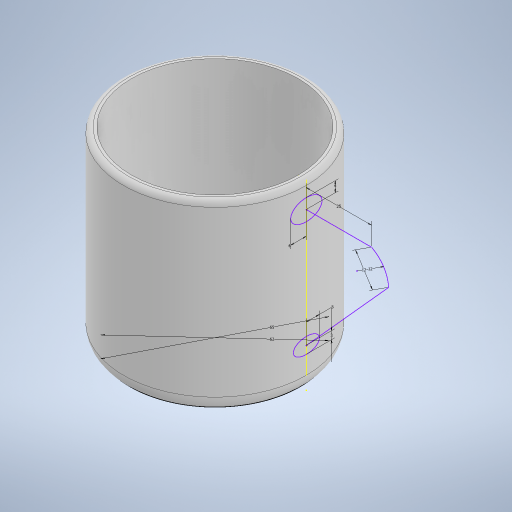
# Autodesk Inventor part: Taza Juan Molina
Saved by Autodesk Inventor 2024 (Build 280153000, 153)
## iProperties
Created: 2024-02-24
Part Number: Taza Juan Molina
Material: Genérico
Document SubType Name: Modeling
Designer: jlmol
Density: 1 g/cm^3
Appearance: Valor por defecto
Author: jlmol
Autodesk Inventor part; units mm, degrees
ref_plane "XZ Plane" through (0, 0, 0) normal (0, 1, 0) x (-1, 0, 0)
sketch "Boceto1" plane through (0, 0, 0) normal (0, 0, 1) x (1, 0, 0)
  line L0 (0, 0) -> (-32.5, 0)
  line L1 (0, 0) -> (0, 70)
  line L2 (0, 70) -> (-35, 70)
  line L3 (-35, 70) -> (-35, 5)
  arc A0 (-35, 5) -> (-32.5, 0) centre (-28.75, 5) ccw
  dimension "d0" = 32.5
  dimension "d1" = 70
  dimension "d2" = 35
  dimension "d3" = 65
  constraints: 8 end point, 2 perpendicular, 2 point on circle, 1 centre point, 1 horizontal, 1 tangent, 1 vertical
  measures "d0" distance of L0.start L0.end
  measures "d1" distance of L0.start L1.end
  measures "d2" distance of L1.end L2.end
  measures "d3" distance of L2.end L3.end
revolve "Revolución1" add sketch "Boceto1" angle 360 about axis through (0, 0, 0) along (0, 1, 0)
shell "Vaciado1" thickness 3 removed faces 1 at (-0.2748, 70, -9.3581)
sketch "Boceto2" plane through (0, 0, 0) normal (0, 0, 1) x (1, 0, 0)
  line L0 (35, 5) -> (35, 70) projected
  line L1 (32, 5) -> (32, 70) projected
  line L2 (35, 60.0697) -> (60, 60.0697)
  arc A0 (66.5079, 49.9877) -> (60, 60.0697) centre (54.5227, 49.3927) ccw
  line L3 (66.5079, 49.9877) -> (35, 15)
  point P0 (0, 0)
  dimension "d10" = 25
  dimension "d11" = 12
  dimension "d12" = 12
  constraints: 4 end point, 2 point on circle, 2 point on line, 1 centre point, 1 horizontal
  measures "d10" distance of L2.start L2.end
  measures "d11" distance of L2.end L3.start
  measures "d12" radius of A0
ref_plane "Plano de trabajo1" through (35, 60.0697, 0) normal (1, 0, 0) x (0, 1, 0)
sketch "Boceto3" plane through (35, 60.0697, 0) normal (1, 0, 0) x (0, 1, 0)
  ellipse E0 centre (0, 0) end of major axis (-4, 0) minor radius 6
  point P0 (-60.0697, 0)
  dimension "d14" = 4
  dimension "d15" = 6
  constraints: 2 other
ref_plane "Plano de trabajo10" through (35, 15, 0) normal (1, 0, 0) x (0, 1, 0)
sketch "Boceto8" plane through (35, 15, 0) normal (1, 0, 0) x (0, 1, 0)
  ellipse E0 centre (0, 0) end of major axis (-3, 0) minor radius 5
  point P0 (-15, 0)
  dimension "d23" = 5
  dimension "d24" = 3
  constraints: 2 other
fillet "Empalme1" radius 2 1 edges at (35, 70, 0)
sketch "Boceto9" plane through (0, 0, 0) normal (0, -1, 0) x (1, 0, 0)
  circle A0 centre (0, 0) radius 32.5
  circle A1 centre (0, 0) radius 31
  dimension "d26" = 65
  dimension "d27" = 62
  constraints: 2 centre point, 2 coincident
  measures "d26" diameter of A0
  measures "d27" diameter of A1
